Autodesk Inventor part; units mm, degrees
(part 2 of 2)
extrude "Extrusion73" add sketch "Sketch81" against normal up to surface (114.1392 mm away)
sketch "Sketch82" plane through (16, -38.25, 43.0952) normal (1, 0, 0) x (0, 0, -1)
  line L0 (81.9898, 142.6892) -> (81.9898, 132.6892) projected
  line L1 (82.5957, 28.55) -> (82.5957, 142.6892) projected
  line L2 (81.9898, 142.6892) -> (82.5957, 142.6892)
  line L3 (82.5957, 142.6892) -> (82.5957, 132.6892)
  line L4 (82.5957, 132.6892) -> (81.9898, 132.6892)
  line L5 (81.9898, 132.6892) -> (81.9898, 142.6892)
  line L6 (81.9898, 132.6892) -> (0, 132.6892) projected
  point P0 (43.0952, 38.25)
  point P1 (82.5957, 142.6892)
  point P2 (81.9898, 132.6892)
  dimension "d460" = 0
  constraints: 8 end point, 2 parallel, 1 horizontal, 1 perpendicular, 1 point on line
  measures "d460" distance between parallel lines of L4 L6
extrude "Extrusion74" add sketch "Sketch82" along normal up to surface (89 mm away)
sketch "Sketch83" plane through (0, 104.4392, 43.0952) normal (0, 1, 0) x (1, 0, 0)
  line L0 (0, 82.5957) -> (0, 0) projected
  line L1 (0, 0) -> (105, 0)
  line L2 (105, 0) -> (105, 3.595)
  line L3 (105, 3.595) -> (0, 3.595)
  line L4 (0, 3.595) -> (0, 0)
  line L5 (105, 0) -> (105, 82.5957) projected
  point P0 (0, 43.0952)
  dimension "d463" = 0
  dimension "d464" = 3.595
  constraints: 8 end point, 2 parallel, 1 horizontal, 1 perpendicular
  measures "d463" distance between parallel lines of L5 L2
  measures "d464" distance of L1.end L2.end
extrude "Extrusion75" cut sketch "Sketch83" against normal up to surface (142.6892 mm away)
sketch "Sketch84" plane through (105, 94.4392, -39.5005) normal (1, 0, 0) x (0, 0, -1)
  line L0 (0, -104.1392) -> (-24.0005, -104.1392) projected
  line L1 (-79.0007, 10) -> (0, 10) projected
  line L2 (0, -104.1392) -> (-0.828, -104.1392)
  line L3 (-0.828, -104.1392) -> (-0.828, 10)
  line L4 (-0.828, 10) -> (0, 10)
  line L5 (0, 10) -> (0, -104.1392)
  point P0 (-39.5005, -94.4392)
  point P1 (-0.828, -104.1392)
  dimension "d468" = 0.828
  constraints: 8 end point, 2 parallel, 1 horizontal, 1 perpendicular, 1 point on line
  measures "d468" distance between parallel lines of L5 L3
extrude "Extrusion76" cut sketch "Sketch84" against normal up to surface (105 mm away)
sketch "Sketch85" plane through (105, 94.4392, 39.5002) normal (1, 0, 0) x (0, 0, -1)
  line L0 (21.1, -132.6892) -> (0, -132.6892) projected
  line L1 (78.1727, 10) -> (0, 10) projected
  line L2 (0, -132.6892) -> (0.173, -132.6892)
  line L3 (0.173, -132.6892) -> (0.173, 10)
  line L4 (0.173, 10) -> (0, 10)
  line L5 (0, 10) -> (0, -132.6892)
  point P0 (39.5002, -94.4392)
  dimension "d471" = 0.173
  constraints: 8 end point, 2 parallel, 1 horizontal, 1 perpendicular, 1 point on line
  measures "d471" distance between parallel lines of L5 L3
extrude "Extrusion77" cut sketch "Sketch85" against normal up to surface (105 mm away)
body "Solid1"
